Autodesk Inventor part; units mm, degrees
(part 2 of 2)
sketch "Sketch8" plane through (0, 0, 6.35) normal (0, 0, 1) x (1, 0, 0)
  line L0 (104.7603, 38.0935) -> (104.7603, 31.7435) projected
  line L1 (104.7603, 31.7435) -> (59.5313, 31.7435) projected
  line L2 (59.5312, 44.45) -> (59.5312, -43.1165) projected
  line L3 (60.2257, -17.7281) -> (66.5757, -17.7281) projected
  line L4 (66.5757, -17.7281) -> (66.5757, -24.0781) projected
  line L5 (59.5312, -43.1165) -> (168.3012, -43.1165) projected
  line L6 (72.9257, -24.0781) -> (72.9257, -17.7281) projected
  line L7 (72.9257, -17.7281) -> (79.2757, -17.7281) projected
  line L8 (79.2757, -17.7281) -> (79.2757, -24.0781) projected
  line L9 (59.5312, -43.1165) -> (168.3012, -43.1165) projected
  line L10 (85.6257, -24.0781) -> (85.6257, -17.7281) projected
  line L11 (85.6257, -17.7281) -> (91.9757, -17.7281) projected
  line L12 (91.9757, -17.7281) -> (91.9757, -24.0781) projected
  line L13 (59.5312, -43.1165) -> (168.3012, -43.1165) projected
  line L14 (98.3257, -24.0781) -> (98.3257, -17.7281) projected
  line L15 (98.3257, -17.7281) -> (104.6757, -17.7281) projected
  line L16 (104.6757, -17.7281) -> (104.6757, -24.0781) projected
  line L17 (59.5312, -43.1165) -> (168.3012, -43.1165) projected
  line L18 (111.0257, -24.0781) -> (111.0257, -17.7281) projected
  line L19 (111.0257, -17.7281) -> (117.3757, -17.7281) projected
  line L20 (117.3757, -17.7281) -> (117.3757, -24.0781) projected
  line L21 (59.5312, -43.1165) -> (168.3012, -43.1165) projected
  line L22 (123.7257, -24.0781) -> (123.7257, -17.7281) projected
  line L23 (123.7257, -17.7281) -> (130.0757, -17.7281) projected
  line L24 (130.0757, -17.7281) -> (130.0757, -24.0781) projected
  line L25 (59.5312, -43.1165) -> (168.3012, -43.1165) projected
  line L26 (136.4257, -24.0781) -> (136.4257, -17.7281) projected
  line L27 (136.4257, -17.7281) -> (66.5757, -17.7281) projected
  line L28 (142.8603, -36.7665) -> (142.8603, -43.1165) projected
  arc A0 (167.6347, -14.6661) -> (167.794, -12.7147) centre (0, 0) ccw projected
  arc A1 (167.794, -12.7147) -> (173.6338, -11.127) centre (160.9087, 24.1445) ccw projected
  arc A2 (173.6338, -11.127) -> (173.7516, -9.1059) centre (0, 0) ccw projected
  arc A3 (173.7516, -9.1059) -> (168.1355, -6.851) centre (157.0177, -42.6616) ccw projected
  arc A4 (168.1355, -6.851) -> (168.2038, -4.8942) centre (0, 0) ccw projected
  arc A5 (168.2038, -4.8942) -> (173.9635, -3.0365) centre (159.6111, 31.6047) ccw projected
  arc A6 (173.9635, -3.0365) -> (173.9871, -1.0122) centre (0, 0) ccw projected
  arc A7 (173.9871, -1.0122) -> (168.2722, 0.979) centre (158.8325, -35.3101) ccw projected
  arc A8 (168.2722, 0.979) -> (168.2494, 2.9368) centre (0, 0) ccw projected
  arc A9 (168.2494, 2.9368) -> (173.9164, 5.0605) centre (157.9679, 38.9964) ccw projected
  arc A10 (173.9164, 5.0605) -> (173.8457, 7.0837) centre (0, 0) ccw projected
  arc A11 (173.8457, 7.0837) -> (168.0444, 8.8068) centre (160.3033, -27.8822) ccw projected
  arc A12 (168.0444, 8.8068) -> (167.9305, 10.7615) centre (0, 0) ccw projected
  arc A13 (167.9305, 10.7615) -> (173.4926, 13.1465) centre (155.9825, 46.3037) ccw projected
  arc A14 (173.4926, 13.1465) -> (173.3279, 15.1642) centre (0, 0) ccw projected
  arc A15 (173.3279, 15.1642) -> (167.4527, 16.6156) centre (161.427, -20.3938) ccw projected
  arc A16 (167.4527, 16.6156) -> (167.248, 18.5628) centre (0, 0) ccw projected
  arc A17 (167.248, 18.5628) -> (172.6931, 21.204) centre (153.6593, 53.5107) ccw projected
  arc A18 (172.6931, 21.204) -> (172.4347, 23.2119) centre (0, 0) ccw projected
  arc A19 (172.4347, 23.2119) -> (166.4983, 24.3884) centre (162.201, -12.8613) ccw projected
  arc A20 (166.4983, 24.3884) -> (166.2033, 26.324) centre (0, 0) ccw projected
  arc A21 (166.2033, 26.324) -> (171.5196, 29.2157) centre (151.0033, 60.6018) ccw projected
  arc A22 (171.5196, 29.2157) -> (171.168, 31.2094) centre (0, 0) ccw projected
  arc A23 (171.168, 31.2094) -> (165.1833, 32.1084) centre (162.6237, -5.3009) ccw projected
  arc A24 (165.1833, 32.1084) -> (164.7985, 34.0282) centre (0, 0) ccw projected
  arc A25 (164.7985, 34.0282) -> (169.9746, 37.1641) centre (148.0203, 67.5617) ccw projected
  arc A26 (169.9746, 37.1641) -> (169.5306, 39.1392) centre (0, 0) ccw projected
  arc A27 (169.5306, 39.1392) -> (163.5106, 39.7588) centre (162.6942, 2.271) ccw projected
  arc A28 (163.5106, 39.7588) -> (163.0369, 41.6586) centre (0, 0) ccw projected
  arc A29 (163.0369, 41.6586) -> (168.0614, 45.0319) centre (144.7166, 74.3752) ccw projected
  arc A30 (168.0614, 45.0319) -> (167.5261, 46.9843) centre (0, 0) ccw projected
  arc A31 (167.5261, 46.9843) -> (161.4837, 47.3231) centre (162.4124, 9.8379) ccw projected
  arc A32 (161.4837, 47.3231) -> (160.9222, 49.1988) centre (0, 0) ccw projected
  arc A33 (160.9222, 49.1988) -> (165.7843, 52.8023) centre (141.0996, 81.0276) ccw projected
  arc A34 (165.7843, 52.8023) -> (165.1587, 54.7276) centre (0, 0) ccw projected
  arc A35 (165.1587, 54.7276) -> (159.1071, 54.785) centre (161.7788, 17.3835) ccw projected
  arc A36 (159.1071, 54.785) -> (158.4589, 56.6325) centre (0, 0) ccw projected
  arc A37 (158.4589, 56.6325) -> (163.1482, 60.4583) centre (137.177, 87.5046) ccw projected
  arc A38 (163.1482, 60.4583) -> (162.4337, 62.3524) centre (0, 0) ccw projected
  arc A39 (162.4337, 62.3524) -> (156.386, 62.1282) centre (160.7949, 24.8915) ccw projected
  arc A40 (156.386, 62.1282) -> (155.6525, 63.9436) centre (0, 0) ccw projected
  arc A41 (155.6525, 63.9436) -> (160.1586, 67.9833) centre (132.9572, 93.792) ccw projected
  arc A42 (160.1586, 67.9833) -> (159.3568, 69.8422) centre (0, 0) ccw projected
  arc A43 (159.3568, 69.8422) -> (153.3261, 69.3368) centre (159.4627, 32.3456) ccw projected
  arc A44 (153.3261, 69.3368) -> (152.5089, 71.1161) centre (0, 0) ccw projected
  arc A45 (152.5089, 71.1161) -> (156.8223, 75.3611) centre (128.4496, 99.8763) ccw projected
  arc A46 (156.8223, 75.3611) -> (155.9348, 77.1807) centre (0, 0) ccw projected
  arc A47 (155.9348, 77.1807) -> (149.9341, 76.3953) centre (157.7851, 39.7296) ccw projected
  arc A48 (149.9341, 76.3953) -> (149.0351, 78.1346) centre (0, 0) ccw projected
  arc A49 (149.0351, 78.1346) -> (153.1462, 82.5757) centre (123.6637, 105.7443) ccw projected
  arc A50 (153.1462, 82.5757) -> (152.1751, 84.352) centre (0, 0) ccw projected
  arc A51 (152.1751, 84.352) -> (146.2174, 83.2883) centre (155.7658, 47.0276) ccw projected
  arc A52 (146.2174, 83.2883) -> (145.2385, 84.9839) centre (0, 0) ccw projected
  arc A53 (145.2385, 84.9839) -> (149.1385, 89.6115) centre (118.61, 111.3833) ccw projected
  arc A54 (149.1385, 89.6115) -> (148.0858, 91.3407) centre (0, 0) ccw projected
  arc A55 (148.0858, 91.3407) -> (142.1841, 90.0009) centre (153.4091, 54.2237) ccw projected
  arc A56 (142.1841, 90.0009) -> (141.1273, 91.6491) centre (0, 0) ccw projected
  arc A57 (141.1273, 91.6491) -> (144.8078, 96.4532) centre (113.2994, 116.7811) ccw projected
  arc A58 (144.8078, 96.4532) -> (143.6758, 98.1315) centre (0, 0) ccw projected
  arc A59 (143.6758, 98.1315) -> (137.8428, 96.5186) centre (150.7202, 61.3024) ccw projected
  arc A60 (137.8428, 96.5186) -> (136.7105, 98.1159) centre (0, 0) ccw projected
  arc A61 (136.7105, 98.1159) -> (140.1635, 103.0859) centre (107.7434, 121.9259) ccw projected
  arc A62 (140.1635, 103.0859) -> (138.9546, 104.7098) centre (0, 0) ccw projected
  arc A63 (138.9546, 104.7098) -> (133.203, 102.8272) centre (147.7049, 68.2483) ccw projected
  arc A64 (133.203, 102.8272) -> (131.9975, 104.3701) centre (0, 0) ccw projected
  arc A65 (131.9975, 104.3701) -> (135.2156, 109.4955) centre (101.9541, 126.8067) ccw projected
  arc A66 (135.2156, 109.4955) -> (133.9325, 111.0613) centre (0, 0) ccw projected
  arc A67 (133.9325, 111.0613) -> (128.2747, 108.9132) centre (144.3697, 75.0464) ccw projected
  arc A68 (128.2747, 108.9132) -> (126.9988, 110.3983) centre (0, 0) ccw projected
  arc A69 (126.9988, 110.3983) -> (129.9749, 115.6678) centre (95.944, 131.4128) ccw projected
  arc A70 (129.9749, 115.6678) -> (128.6203, 117.1723) centre (0, 0) ccw projected
  arc A71 (128.6203, 117.1723) -> (123.0685, 114.7633) centre (140.7218, 81.682) ccw projected
  arc A72 (123.0685, 114.7633) -> (121.7249, 116.1874) centre (0, 0) ccw projected
  arc A73 (121.7249, 116.1874) -> (124.4527, 121.5897) centre (89.7261, 135.7343) ccw projected
  arc A74 (124.4527, 121.5897) -> (123.0295, 123.0295) centre (0, 0) ccw projected
  arc A75 (123.0295, 123.0295) -> (117.5959, 120.3648) centre (136.7691, 88.1407) ccw projected
  arc A76 (117.5959, 120.3648) -> (116.1874, 121.7249) centre (0, 0) ccw projected
  arc A77 (116.1874, 121.7249) -> (118.6609, 127.2482) centre (83.3138, 139.7619) ccw projected
  arc A78 (118.6609, 127.2482) -> (117.1723, 128.6203) centre (0, 0) ccw projected
  arc A79 (117.1723, 128.6203) -> (111.8685, 125.7056) centre (132.5202, 94.4085) ccw projected
  arc A80 (111.8685, 125.7056) -> (110.3983, 126.9988) centre (0, 0) ccw projected
  arc A81 (110.3983, 126.9988) -> (112.6121, 132.6312) centre (76.7211, 143.4867) ccw projected
  arc A82 (112.6121, 132.6312) -> (111.0613, 133.9325) centre (0, 0) ccw projected
  arc A83 (111.0613, 133.9325) -> (105.8989, 130.7742) centre (127.9844, 100.4718) ccw projected
  arc A84 (105.8989, 130.7742) -> (104.3701, 131.9975) centre (0, 0) ccw projected
  arc A85 (104.3701, 131.9975) -> (106.3195, 137.7269) centre (69.9623, 146.9008) ccw projected
  arc A86 (106.3195, 137.7269) -> (104.7098, 138.9546) centre (0, 0) ccw projected
  arc A87 (104.7098, 138.9546) -> (99.6999, 135.5596) centre (123.1713, 106.3175) ccw projected
  arc A88 (99.6999, 135.5596) -> (98.1159, 136.7105) centre (0, 0) ccw projected
  arc A89 (98.1159, 136.7105) -> (99.7966, 142.5243) centre (63.0519, 149.9968) ccw projected
  arc A90 (99.7966, 142.5243) -> (98.1315, 143.6758) centre (0, 0) ccw projected
  arc A91 (98.1315, 143.6758) -> (93.285, 140.0514) centre (118.0914, 111.933) ccw projected
  arc A92 (93.285, 140.0514) -> (91.6491, 141.1273) centre (0, 0) ccw projected
  arc A93 (91.6491, 141.1273) -> (93.0575, 147.013) centre (56.005, 152.7678) ccw projected
  arc A94 (93.0575, 147.013) -> (91.3407, 148.0858) centre (0, 0) ccw projected
  arc A95 (91.3407, 148.0858) -> (86.668, 144.2398) centre (112.7558, 117.306) ccw projected
  arc A96 (86.668, 144.2398) -> (84.9839, 145.2385) centre (0, 0) ccw projected
  arc A97 (84.9839, 145.2385) -> (86.1169, 151.1833) centre (48.8368, 155.2081) ccw projected
  arc A98 (86.1169, 151.1833) -> (84.352, 152.1751) centre (0, 0) ccw projected
  arc A99 (84.352, 152.1751) -> (79.8634, 148.1159) centre (107.176, 122.425) ccw projected
  arc A100 (79.8634, 148.1159) -> (78.1346, 149.0351) centre (0, 0) ccw projected
  arc A101 (78.1346, 149.0351) -> (78.9898, 155.0262) centre (41.5628, 157.3121) ccw projected
  arc A102 (78.9898, 155.0262) -> (77.1807, 155.9348) centre (0, 0) ccw projected
  arc A103 (77.1807, 155.9348) -> (72.8858, 151.6712) centre (101.3641, 127.2788) ccw projected
  arc A104 (72.8858, 151.6712) -> (71.1161, 152.5089) centre (0, 0) ccw projected
  arc A105 (71.1161, 152.5089) -> (71.6916, 158.5334) centre (34.1988, 159.0755) ccw projected
  arc A106 (71.6916, 158.5334) -> (69.8422, 159.3568) centre (0, 0) ccw projected
  arc A107 (69.8422, 159.3568) -> (65.7503, 154.898) centre (95.3327, 131.857) ccw projected
  arc A108 (65.7503, 154.898) -> (63.9436, 155.6525) centre (0, 0) ccw projected
  arc A109 (63.9436, 155.6525) -> (64.2382, 161.6972) centre (26.7607, 160.4944) ccw projected
  arc A110 (64.2382, 161.6972) -> (62.3524, 162.4337) centre (0, 0) ccw projected
  arc A111 (62.3524, 162.4337) -> (58.4724, 157.7893) centre (89.0948, 136.1495) ccw projected
  arc A112 (58.4724, 157.7893) -> (56.6325, 158.4589) centre (0, 0) ccw projected
  arc A113 (56.6325, 158.4589) -> (56.6456, 164.5108) centre (19.2647, 161.5656) ccw projected
  arc A114 (56.6456, 164.5108) -> (54.7276, 165.1587) centre (0, 0) ccw projected
  arc A115 (54.7276, 165.1587) -> (51.0679, 160.3388) centre (82.6639, 140.1473) ccw projected
  arc A116 (51.0679, 160.3388) -> (49.1988, 160.9222) centre (0, 0) ccw projected
  arc A117 (49.1988, 160.9222) -> (48.9303, 166.9681) centre (11.7269, 162.2869) ccw projected
  arc A118 (48.9303, 166.9681) -> (46.9843, 167.5261) centre (0, 0) ccw projected
  arc A119 (46.9843, 167.5261) -> (43.5528, 162.5412) centre (76.054, 143.8415) ccw projected
  arc A120 (43.5528, 162.5412) -> (41.6586, 163.0369) centre (0, 0) ccw projected
  arc A121 (41.6586, 163.0369) -> (41.1091, 169.0638) centre (4.1638, 162.6568) ccw projected
  arc A122 (41.1091, 169.0638) -> (39.1392, 169.5306) centre (0, 0) ccw projected
  arc A123 (39.1392, 169.5306) -> (35.9433, 164.3915) centre (69.2793, 147.2241) ccw projected
  arc A124 (35.9433, 164.3915) -> (34.0282, 164.7985) centre (0, 0) ccw projected
  arc A125 (34.0282, 164.7985) -> (33.1989, 170.7933) centre (-3.4084, 162.6744) ccw projected
  arc A126 (33.1989, 170.7933) -> (31.2094, 171.168) centre (0, 0) ccw projected
  arc A127 (31.2094, 171.168) -> (28.256, 165.8857) centre (62.3547, 150.288) ccw projected
  arc A128 (28.256, 165.8857) -> (26.324, 166.2033) centre (0, 0) ccw projected
  arc A129 (26.324, 166.2033) -> (25.2167, 172.153) centre (-10.9732, 162.3397) ccw projected
  arc A130 (25.2167, 172.153) -> (23.2119, 172.4347) centre (0, 0) ccw projected
  arc A131 (23.2119, 172.4347) -> (20.5076, 167.0207) centre (55.295, 153.0263) ccw projected
  arc A132 (20.5076, 167.0207) -> (18.5628, 167.248) centre (0, 0) ccw projected
  arc A133 (18.5628, 167.248) -> (17.1799, 173.1397) centre (-18.5142, 161.6533) ccw projected
  arc A134 (17.1799, 173.1397) -> (15.1642, 173.3279) centre (0, 0) ccw projected
  arc A135 (15.1642, 173.3279) -> (12.7147, 167.794) centre (48.1155, 155.4332) ccw projected
  arc A136 (12.7147, 167.794) -> (10.7615, 167.9305) centre (0, 0) ccw projected
  arc A137 (10.7615, 167.9305) -> (9.1059, 173.7516) centre (-26.0151, 160.6169) ccw projected
  arc A138 (9.1059, 173.7516) -> (7.0837, 173.8457) centre (0, 0) ccw projected
  arc A139 (7.0837, 173.8457) -> (4.8942, 168.2038) centre (40.8318, 157.5035) ccw projected
  arc A140 (4.8942, 168.2038) -> (2.9368, 168.2494) centre (0, 0) ccw projected
  arc A141 (2.9368, 168.2494) -> (1.0122, 173.9871) centre (-33.4597, 159.2326) ccw projected
  arc A142 (1.0122, 173.9871) -> (-1.0122, 173.9871) centre (0, 0) ccw projected
  arc A143 (-1.0122, 173.9871) -> (-2.9368, 168.2494) centre (33.4597, 159.2326) ccw projected
  arc A144 (-2.9368, 168.2494) -> (-4.8942, 168.2038) centre (0, 0) ccw projected
  arc A145 (-4.8942, 168.2038) -> (-7.0837, 173.8457) centre (-40.8318, 157.5035) ccw projected
  arc A146 (-7.0837, 173.8457) -> (-118.6609, 127.2482) centre (0, 0) ccw projected
  arc A147 (-118.6609, 127.2482) -> (-116.1874, 121.7249) centre (-83.3138, 139.7619) ccw projected
  arc A148 (-116.1874, 121.7249) -> (-117.5959, 120.3648) centre (0, 0) ccw projected
  arc A149 (-117.5959, 120.3648) -> (-123.0295, 123.0295) centre (-136.7691, 88.1407) ccw projected
  arc A150 (-123.0295, 123.0295) -> (-124.4527, 121.5897) centre (0, 0) ccw projected
  arc A151 (-124.4527, 121.5897) -> (-121.7249, 116.1874) centre (-89.7261, 135.7343) ccw projected
  arc A152 (-121.7249, 116.1874) -> (-123.0685, 114.7633) centre (0, 0) ccw projected
  arc A153 (-123.0685, 114.7633) -> (-128.6203, 117.1723) centre (-140.7218, 81.682) ccw projected
  arc A154 (-128.6203, 117.1723) -> (-129.9749, 115.6678) centre (0, 0) ccw projected
  arc A155 (-129.9749, 115.6678) -> (-126.9988, 110.3983) centre (-95.944, 131.4128) ccw projected
  arc A156 (-126.9988, 110.3983) -> (-128.2747, 108.9132) centre (0, 0) ccw projected
  arc A157 (-128.2747, 108.9132) -> (-133.9325, 111.0613) centre (-144.3697, 75.0464) ccw projected
  arc A158 (-133.9325, 111.0613) -> (-135.2156, 109.4955) centre (0, 0) ccw projected
  arc A159 (-135.2156, 109.4955) -> (-131.9975, 104.3701) centre (-101.9541, 126.8067) ccw projected
  arc A160 (-131.9975, 104.3701) -> (-133.203, 102.8272) centre (0, 0) ccw projected
  arc A161 (-133.203, 102.8272) -> (-138.9546, 104.7098) centre (-147.7049, 68.2483) ccw projected
  arc A162 (-138.9546, 104.7098) -> (-140.1635, 103.0859) centre (0, 0) ccw projected
  arc A163 (-140.1635, 103.0859) -> (-136.7105, 98.1159) centre (-107.7434, 121.9259) ccw projected
  arc A164 (-136.7105, 98.1159) -> (-137.8428, 96.5186) centre (0, 0) ccw projected
  arc A165 (-137.8428, 96.5186) -> (-143.6758, 98.1315) centre (-150.7202, 61.3024) ccw projected
  arc A166 (-143.6758, 98.1315) -> (-144.8078, 96.4532) centre (0, 0) ccw projected
  arc A167 (-144.8078, 96.4532) -> (-141.1273, 91.6491) centre (-113.2994, 116.7811) ccw projected
  arc A168 (-141.1273, 91.6491) -> (-142.1841, 90.0009) centre (0, 0) ccw projected
  arc A169 (-142.1841, 90.0009) -> (-148.0858, 91.3407) centre (-153.4091, 54.2237) ccw projected
  arc A170 (-148.0858, 91.3407) -> (-149.1385, 89.6115) centre (0, 0) ccw projected
  arc A171 (-149.1385, 89.6115) -> (-145.2385, 84.9839) centre (-118.61, 111.3833) ccw projected
  arc A172 (-145.2385, 84.9839) -> (-146.2174, 83.2883) centre (0, 0) ccw projected
  arc A173 (-146.2174, 83.2883) -> (-152.1751, 84.352) centre (-155.7658, 47.0276) ccw projected
  arc A174 (-152.1751, 84.352) -> (-153.1462, 82.5757) centre (0, 0) ccw projected
  arc A175 (-153.1462, 82.5757) -> (-149.0351, 78.1346) centre (-123.6637, 105.7443) ccw projected
  arc A176 (-149.0351, 78.1346) -> (-149.9341, 76.3953) centre (0, 0) ccw projected
  arc A177 (-149.9341, 76.3953) -> (-155.9348, 77.1807) centre (-157.7851, 39.7296) ccw projected
  arc A178 (-155.9348, 77.1807) -> (-156.8223, 75.3611) centre (0, 0) ccw projected
  arc A179 (-156.8223, 75.3611) -> (-152.5089, 71.1161) centre (-128.4496, 99.8763) ccw projected
  arc A180 (-152.5089, 71.1161) -> (-153.3261, 69.3368) centre (0, 0) ccw projected
  arc A181 (-153.3261, 69.3368) -> (-159.3568, 69.8422) centre (-159.4627, 32.3456) ccw projected
  arc A182 (-159.3568, 69.8422) -> (-160.1586, 67.9833) centre (0, 0) ccw projected
  arc A183 (-160.1586, 67.9833) -> (-155.6525, 63.9436) centre (-132.9572, 93.792) ccw projected
  arc A184 (-155.6525, 63.9436) -> (-156.386, 62.1282) centre (0, 0) ccw projected
  arc A185 (-156.386, 62.1282) -> (-162.4337, 62.3524) centre (-160.7949, 24.8915) ccw projected
  arc A186 (-162.4337, 62.3524) -> (-163.1482, 60.4583) centre (0, 0) ccw projected
  arc A187 (-163.1482, 60.4583) -> (-158.4589, 56.6325) centre (-137.177, 87.5046) ccw projected
  arc A188 (-158.4589, 56.6325) -> (-159.1071, 54.785) centre (0, 0) ccw projected
  arc A189 (-159.1071, 54.785) -> (-165.1587, 54.7276) centre (-161.7788, 17.3835) ccw projected
  arc A190 (-165.1587, 54.7276) -> (-165.7843, 52.8023) centre (0, 0) ccw projected
  arc A191 (-165.7843, 52.8023) -> (-160.9222, 49.1988) centre (-141.0996, 81.0276) ccw projected
  arc A192 (-160.9222, 49.1988) -> (-161.4837, 47.3231) centre (0, 0) ccw projected
  arc A193 (-161.4837, 47.3231) -> (-167.5261, 46.9843) centre (-162.4124, 9.8379) ccw projected
  arc A194 (-167.5261, 46.9843) -> (-168.0614, 45.0319) centre (0, 0) ccw projected
  arc A195 (-168.0614, 45.0319) -> (-163.0369, 41.6586) centre (-144.7166, 74.3752) ccw projected
  arc A196 (-163.0369, 41.6586) -> (-163.5106, 39.7588) centre (0, 0) ccw projected
  arc A197 (-163.5106, 39.7588) -> (-169.5306, 39.1392) centre (-162.6942, 2.271) ccw projected
  arc A198 (-169.5306, 39.1392) -> (-169.9746, 37.1641) centre (0, 0) ccw projected
  arc A199 (-169.9746, 37.1641) -> (-164.7985, 34.0282) centre (-148.0203, 67.5617) ccw projected
  arc A200 (-164.7985, 34.0282) -> (-165.1833, 32.1084) centre (0, 0) ccw projected
  arc A201 (-165.1833, 32.1084) -> (-171.168, 31.2094) centre (-162.6237, -5.3009) ccw projected
  arc A202 (-171.168, 31.2094) -> (-171.5196, 29.2157) centre (0, 0) ccw projected
  arc A203 (-171.5196, 29.2157) -> (-166.2033, 26.324) centre (-151.0033, 60.6018) ccw projected
  arc A204 (-166.2033, 26.324) -> (-166.4983, 24.3884) centre (0, 0) ccw projected
  arc A205 (-166.4983, 24.3884) -> (-172.4347, 23.2119) centre (-162.201, -12.8613) ccw projected
  arc A206 (-172.4347, 23.2119) -> (-172.6931, 21.204) centre (0, 0) ccw projected
  arc A207 (-172.6931, 21.204) -> (-167.248, 18.5628) centre (-153.6593, 53.5107) ccw projected
  arc A208 (-167.248, 18.5628) -> (-167.4527, 16.6156) centre (0, 0) ccw projected
  arc A209 (-167.4527, 16.6156) -> (-173.3279, 15.1642) centre (-161.427, -20.3938) ccw projected
  arc A210 (-173.3279, 15.1642) -> (-173.4926, 13.1465) centre (0, 0) ccw projected
  arc A211 (-173.4926, 13.1465) -> (-167.9305, 10.7615) centre (-155.9825, 46.3037) ccw projected
  arc A212 (-167.9305, 10.7615) -> (-168.0444, 8.8068) centre (0, 0) ccw projected
  arc A213 (-168.0444, 8.8068) -> (-173.8457, 7.0837) centre (-160.3033, -27.8822) ccw projected
  arc A214 (-173.8457, 7.0837) -> (-173.9164, 5.0605) centre (0, 0) ccw projected
  arc A215 (-173.9164, 5.0605) -> (-168.2494, 2.9368) centre (-157.9679, 38.9964) ccw projected
  arc A216 (-168.2494, 2.9368) -> (-168.2722, 0.979) centre (0, 0) ccw projected
  arc A217 (-168.2722, 0.979) -> (-173.9871, -1.0122) centre (-158.8325, -35.3101) ccw projected
  arc A218 (-173.9871, -1.0122) -> (-173.9635, -3.0365) centre (0, 0) ccw projected
  arc A219 (-173.9635, -3.0365) -> (-168.2038, -4.8942) centre (-159.6111, 31.6047) ccw projected
  arc A220 (-168.2038, -4.8942) -> (-168.1355, -6.851) centre (0, 0) ccw projected
  arc A221 (-168.1355, -6.851) -> (-173.7516, -9.1059) centre (-157.0177, -42.6616) ccw projected
  arc A222 (-173.7516, -9.1059) -> (-173.6338, -11.127) centre (0, 0) ccw projected
  arc A223 (-173.6338, -11.127) -> (-167.794, -12.7147) centre (-160.9087, 24.1445) ccw projected
  arc A224 (-167.794, -12.7147) -> (-167.6347, -14.6661) centre (0, 0) ccw projected
  arc A225 (-167.6347, -14.6661) -> (-173.1397, -17.1799) centre (-154.8628, -49.9207) ccw projected
  arc A226 (-173.1397, -17.1799) -> (-172.9281, -19.1933) centre (0, 0) ccw projected
  arc A227 (-172.9281, -19.1933) -> (-167.0207, -20.5076) centre (-161.8578, 16.632) ccw projected
  arc A228 (-167.0207, -20.5076) -> (-166.7708, -22.4495) centre (0, 0) ccw projected
  arc A229 (-166.7708, -22.4495) -> (-172.153, -25.2167) centre (-152.3726, -57.0717) ccw projected
  arc A230 (-172.153, -25.2167) -> (-171.8479, -27.218) centre (0, 0) ccw projected
  arc A231 (-171.8479, -27.218) -> (-165.8857, -28.256) centre (-162.4563, 9.0836) ccw projected
  arc A232 (-165.8857, -28.256) -> (-165.5457, -30.1843) centre (0, 0) ccw projected
  arc A233 (-165.5457, -30.1843) -> (-170.7933, -33.1989) centre (-149.5523, -64.0991) ccw projected
  arc A234 (-170.7933, -33.1989) -> (-170.3955, -35.1838) centre (0, 0) ccw projected
  arc A235 (-170.3955, -35.1838) -> (-164.3915, -35.9433) centre (-162.703, 1.5154) ccw projected
  arc A236 (-164.3915, -35.9433) -> (-163.9621, -37.8536) centre (0, 0) ccw projected
  arc A237 (-163.9621, -37.8536) -> (-169.0638, -41.1091) centre (-146.4081, -70.9876) ccw projected
  arc A238 (-169.0638, -41.1091) -> (-168.574, -43.0734) centre (0, 0) ccw projected
  arc A239 (-168.574, -43.0734) -> (-168.3012, -43.1165) centre (-162.5974, -6.0561) ccw projected
  arc A240 (-142.7994, 43.3177) -> (-143.3542, 41.4448) centre (0, 0) ccw projected
  arc A241 (-143.3542, 41.4448) -> (-149.3949, 41.0801) centre (-144.1598, 4.5833) ccw projected
  arc A242 (1.0122, 173.9871) -> (-1.0122, 173.9871) centre (0, 0) ccw projected
  arc A243 (-149.9198, 39.121) -> (-144.8708, 35.7848) centre (-127.1377, 68.1106) ccw projected
  arc A244 (-144.8708, 35.7848) -> (-145.3268, 33.8855) centre (0, 0) ccw projected
  arc A245 (-145.3268, 33.8855) -> (-151.3401, 33.2051) centre (-144.2021, -2.9677) ccw projected
  arc A246 (1.0122, 173.9871) -> (-1.0122, 173.9871) centre (0, 0) ccw projected
  arc A247 (-151.7618, 31.2212) -> (-146.5451, 28.1538) centre (-130.5281, 61.3634) ccw projected
  arc A248 (-146.5451, 28.1538) -> (-146.9011, 26.2332) centre (0, 0) ccw projected
  arc A249 (-146.9011, 26.2332) -> (-152.8705, 25.239) centre (-143.8491, -10.5106) ccw projected
  arc A250 (1.0122, 173.9871) -> (-1.0122, 173.9871) centre (0, 0) ccw projected
  arc A251 (-153.1878, 23.2358) -> (-147.8177, 20.4457) centre (-133.5607, 54.448) ccw projected
  arc A252 (-147.8177, 20.4457) -> (-148.0727, 18.509) centre (0, 0) ccw projected
  arc A253 (-148.0727, 18.509) -> (-153.9819, 17.2038) centre (-143.1019, -18.0247) ccw projected
  arc A254 (1.0122, 173.9871) -> (-1.0122, 173.9871) centre (0, 0) ccw projected
  arc A255 (-154.1939, 15.1868) -> (-148.6852, 12.6815) centre (-136.2272, 47.3834) ccw projected
  arc A256 (-148.6852, 12.6815) -> (-148.8384, 10.7342) centre (0, 0) ccw projected
  arc A257 (-148.8384, 10.7342) -> (-154.6713, 9.1214) centre (-141.9624, -25.4894) ccw projected
  arc A258 (1.0122, 173.9871) -> (-1.0122, 173.9871) centre (0, 0) ccw projected
  arc A259 (-154.7774, 7.0961) -> (-149.1451, 4.8825) centre (-138.5204, 40.1889) ccw projected
  arc A260 (-149.1451, 4.8825) -> (-149.1962, 2.9298) centre (0, 0) ccw projected
  arc A261 (-149.1962, 2.9298) -> (-154.9367, 1.0141) centre (-140.4339, -32.8842) ccw projected
  arc A262 (1.0122, 173.9871) -> (-1.0122, 173.9871) centre (0, 0) ccw projected
  arc A263 (-154.9367, -1.0141) -> (-149.1962, -2.9298) centre (-140.4339, 32.8842) ccw projected
  arc A264 (-149.1962, -2.9298) -> (-149.1451, -4.8825) centre (0, 0) ccw projected
  arc A265 (-149.1451, -4.8825) -> (-154.7774, -7.0961) centre (-138.5204, -40.1889) ccw projected
  arc A266 (1.0122, 173.9871) -> (-1.0122, 173.9871) centre (0, 0) ccw projected
  arc A267 (-154.6713, -9.1214) -> (-148.8384, -10.7342) centre (-141.9624, 25.4894) ccw projected
  arc A268 (-148.8384, -10.7342) -> (-148.6852, -12.6815) centre (0, 0) ccw projected
  arc A269 (-148.6852, -12.6815) -> (-154.1939, -15.1868) centre (-136.2272, -47.3834) ccw projected
  arc A270 (1.0122, 173.9871) -> (-1.0122, 173.9871) centre (0, 0) ccw projected
  arc A271 (-153.9819, -17.2038) -> (-148.0727, -18.509) centre (-143.1019, 18.0247) ccw projected
  arc A272 (-148.0727, -18.509) -> (-147.8177, -20.4457) centre (0, 0) ccw projected
  arc A273 (-147.8177, -20.4457) -> (-153.1878, -23.2358) centre (-133.5607, -54.448) ccw projected
  arc A274 (1.0122, 173.9871) -> (-1.0122, 173.9871) centre (0, 0) ccw projected
  arc A275 (-152.8705, -25.239) -> (-146.9011, -26.2332) centre (-143.8491, 10.5106) ccw projected
  arc A276 (-146.9011, -26.2332) -> (-146.5451, -28.1538) centre (0, 0) ccw projected
  arc A277 (-146.5451, -28.1538) -> (-151.7618, -31.2212) centre (-130.5281, -61.3634) ccw projected
  arc A278 (1.0122, 173.9871) -> (-1.0122, 173.9871) centre (0, 0) ccw projected
  arc A279 (-151.3401, -33.2051) -> (-145.3268, -33.8855) centre (-144.2021, 2.9677) ccw projected
  arc A280 (-145.3268, -33.8855) -> (-144.8708, -35.7848) centre (0, 0) ccw projected
  arc A281 (-144.8708, -35.7848) -> (-149.9198, -39.121) centre (-127.1377, -68.1106) ccw projected
  arc A282 (1.0122, 173.9871) -> (-1.0122, 173.9871) centre (0, 0) ccw projected
  arc A283 (-149.3949, -41.0801) -> (-143.3542, -41.4448) centre (-144.1598, -4.5833) ccw projected
  arc A284 (-143.3542, -41.4448) -> (-142.8603, -43.1165) centre (0, 0) ccw projected
  line L29 (-142.8603, -43.1165) -> (-142.8603, -36.7665) projected
  line L30 (-143.5548, -17.7281) -> (-136.4257, -17.7281) projected
  line L31 (-136.4257, -17.7281) -> (-136.4257, -24.0781) projected
  line L32 (59.5312, -43.1165) -> (168.3012, -43.1165) projected
  line L33 (-130.0757, -24.0781) -> (-130.0757, -17.7281) projected
  line L34 (-130.0757, -17.7281) -> (-123.7257, -17.7281) projected
  line L35 (-123.7257, -17.7281) -> (-123.7257, -24.0781) projected
  line L36 (59.5312, -43.1165) -> (168.3012, -43.1165) projected
  line L37 (-117.3757, -24.0781) -> (-117.3757, -17.7281) projected
  line L38 (-117.3757, -17.7281) -> (-111.0257, -17.7281) projected
  line L39 (-111.0257, -17.7281) -> (-111.0257, -24.0781) projected
  line L40 (59.5312, -43.1165) -> (168.3012, -43.1165) projected
  line L41 (-104.6757, -24.0781) -> (-104.6757, -17.7281) projected
  line L42 (-104.6757, -17.7281) -> (-98.3257, -17.7281) projected
  line L43 (-98.3257, -17.7281) -> (-98.3257, -24.0781) projected
  line L44 (59.5312, -43.1165) -> (168.3012, -43.1165) projected
  line L45 (-91.9757, -24.0781) -> (-91.9757, -17.7281) projected
  line L46 (-91.9757, -17.7281) -> (-85.6257, -17.7281) projected
  line L47 (-85.6257, -17.7281) -> (-85.6257, -24.0781) projected
  line L48 (59.5312, -43.1165) -> (168.3012, -43.1165) projected
  line L49 (-79.2757, -24.0781) -> (-79.2757, -17.7281) projected
  line L50 (-79.2757, -17.7281) -> (-72.9257, -17.7281) projected
  line L51 (-72.9257, -17.7281) -> (-72.9257, -24.0781) projected
  line L52 (59.5312, -43.1165) -> (168.3012, -43.1165) projected
  line L53 (-66.5757, -24.0781) -> (-66.5757, -17.7281) projected
  line L54 (-66.5757, -17.7281) -> (-136.4257, -17.7281) projected
  line L55 (-59.5312, -43.1165) -> (-59.5312, 44.45) projected
  line L56 (-59.5313, 31.7435) -> (-104.7603, 31.7435) projected
  line L57 (-104.7603, 31.7435) -> (-104.7603, 38.0935) projected
  line L58 (-104.7603, 38.0935) -> (-59.5313, 38.0935) projected
  line L59 (-59.5312, -43.1165) -> (-59.5312, 44.45) projected
  line L60 (-59.5312, 44.45) -> (-38.1, 44.45) projected
  line L61 (-38.1, 44.45) -> (-38.1, 133.985) projected
  arc A285 (38.1, 133.985) -> (-38.1, 133.985) centre (0, -0.4192) ccw projected
  line L62 (38.1, 133.985) -> (38.1, 44.45) projected
  line L63 (38.1, 44.45) -> (59.5312, 44.45) projected
  line L64 (59.5312, 44.45) -> (59.5312, -43.1165) projected
  line L65 (59.5313, 38.0935) -> (104.7603, 38.0935) projected
  line L66 (-210.1511, -0.4192) -> (214.329, -0.4192)
  point P0 (59.5313, -36.7665)
  point P1 (66.5757, -43.1165)
  point P2 (72.9257, -43.1165)
  point P3 (79.2757, -43.1165)
  point P4 (85.6257, -43.1165)
  point P5 (91.9757, -43.1165)
  point P6 (98.3257, -43.1165)
  point P7 (104.6757, -43.1165)
  point P8 (111.0257, -43.1165)
  point P9 (117.3757, -43.1165)
  point P10 (123.7257, -43.1165)
  point P11 (130.0757, -43.1165)
  point P12 (136.4257, -43.1165)
  point P13 (142.8603, -43.1165)
  point P14 (-136.4257, -43.1165)
  point P15 (-130.0757, -43.1165)
  point P16 (-123.7257, -43.1165)
  point P17 (-117.3757, -43.1165)
  point P18 (-111.0257, -43.1165)
  point P19 (-104.6757, -43.1165)
  point P20 (-98.3257, -43.1165)
  point P21 (-91.9757, -43.1165)
  point P22 (-85.6257, -43.1165)
  point P23 (-79.2757, -43.1165)
  point P24 (-72.9257, -43.1165)
  point P25 (-66.5757, -43.1165)
  point P26 (-59.5313, -36.7665)
  point P27 (60.1157, 31.7565)
  point P28 (-60.1157, 31.7565)
  point P29 (-60.1157, 38.1065)
  point P30 (60.1157, 38.1065)
  point P31 (60.2257, -17.7281)
  point P32 (142.8603, -24.0599)
  point P33 (-142.8603, -24.0599)
  point P34 (-60.2257, -17.7281)
  constraints: 2 end point, 21 other
equation "\"d0\" = da_da"
equation "\"d1\" = da_b"
equation "\"d3\" = da_dw"
equation "\"d15\" = da_aw"
equation "\"d19\" = da_aw"
equation "\"da_da\" = 347.98"
equation "\"da_b\" = 6.35"
equation "\"da_dw\" = 342.9"
equation "\"da_aw\" = 195.58"
body "Solid1"
body "Srf1"
